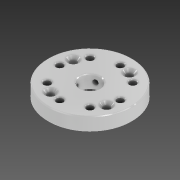
# Autodesk Inventor part: endeffector mount part
Saved by Autodesk Inventor 2020 (Build 240168000, 168)
## iProperties
Created: 2020-05-18
Part Number: endeffector mount part
Material: Generic
Document SubType Name: Modeling
Designer: stefa
Density: 1 g/cm^3
Appearance: Aluminum - Polished
Author: stefa
Autodesk Inventor part; units mm, degrees
ref_plane "YZ Plane" through (0, 0, 0) normal (1, 0, 0) x (0, 1, 0)
ref_plane "XZ Plane" through (0, 0, 0) normal (0, 1, 0) x (-1, 0, 0)
sketch "Sketch1" plane through (0, 0, 0) normal (0, 1, 0) x (-1, 0, 0)
  circle A0 centre (0, 0) radius 6
  circle A1 centre (0, 0) radius 25
  circle A2 centre (0, -18) radius 2
  circle A3 centre (12.7279, -12.7279) radius 2
  circle A4 centre (18, 0) radius 2
  circle A5 centre (12.7279, 12.7279) radius 2
  circle A6 centre (0, 18) radius 2
  circle A7 centre (-12.7279, 12.7279) radius 2
  circle A8 centre (-18, 0) radius 2
  circle A9 centre (-12.7279, -12.7279) radius 2
  circle A10 centre (16.682, -6.761) radius 2
  circle A11 centre (6.761, 16.682) radius 2
  circle A12 centre (-16.682, 6.761) radius 2
  circle A13 centre (-6.761, -16.682) radius 2
  dimension "d0" = 50
  dimension "d1" = 12
  dimension "d4" = 4
  dimension "d5" = 18
  dimension "d8" = 360
  dimension "d18" = 4
  dimension "d21" = 13.7766
  dimension "d22" = 6.8883
  dimension "d23" = 18
  dimension "d26" = 360
  constraints: 14 centre point, 2 coincident, 1 vertical alignment, 26 other
  measures "d0" diameter of A1
  measures "d1" diameter of A0
  measures "d4" diameter of A2
  measures "d5" distance of A2.centre point (0, 0)
  measures "d18" diameter of A10
  measures "d21" distance of A3.centre A4.centre
  measures "d22" distance of A10.centre A4.centre
  measures "d23" distance of A10.centre point (0, 0)
extrude "Extrusion1" add sketch "Sketch1" along normal blind 8
ref_plane "Work Plane2" through (0, 0, 0) normal (0.3826834, 0, 0.9238795) x (0, 1, 0)
sketch "Sketch2" plane through (0, 0, 0) normal (0.3826834, 0, 0.9238795) x (0, 1, 0)
  circle A0 centre (4, 0) radius 1.5
  line L0 (8, -25) -> (8, 25) projected
  line L1 (0, -25) -> (0, 25) projected
  point P0 (0, 0)
  dimension "d11" = 3
  dimension "d12" = 8
  dimension "d13" = 4
  constraints: 1 centre point
  measures "d11" diameter of A0
  measures "d12" distance between parallel lines of L0 L1
  measures "d13" distance from line of A0.centre L0
extrude "Extrusion2" cut sketch "Sketch2" against normal up to surface round surface about axis through (0, 0, 0) along (0, 1, 0) radius 25 far side no
thread "Thread1" size "M3x0.5" class "6H" standard "ANSI Metric M Profile" full length
chamfer "Chamfer1" distance 1.5 angle 45 4 edges at (18.682, 8, 6.761) (-4.761, 8, 16.682) (-14.682, 8, -6.761) (8.761, 8, -16.682)
thread "Thread2" size "M4x0.7" class "6H" standard "ANSI Metric M Profile" full length
thread "Thread3" size "M4x0.7" class "6H" standard "ANSI Metric M Profile" full length
thread "Thread4" size "M4x0.7" class "6H" standard "ANSI Metric M Profile" full length
thread "Thread5" size "M4x0.7" class "6H" standard "ANSI Metric M Profile" full length
thread "Thread6" size "M4x0.7" class "6H" standard "ANSI Metric M Profile" full length
thread "Thread7" size "M4x0.7" class "6H" standard "ANSI Metric M Profile" full length
thread "Thread8" size "M4x0.7" class "6H" standard "ANSI Metric M Profile" full length
thread "Thread9" size "M4x0.7" class "6H" standard "ANSI Metric M Profile" full length
chamfer "Chamfer2" distance 0.5 angle 45 25 edges at (25, 8, 0) (6, 8, 0) (25, 0, 0) (6, 0, 0) (14.7279, 8, -12.7279) (20, 8, 0) (14.7279, 8, 12.7279) (2, 8, 18) (-10.7279, 8, 12.7279) (-16, 8, 0) (-10.7279, 8, -12.7279) (2, 8, -18) (-10.0215, 2.5836, -22.9035) (2, 0, -18) (8.761, 0, -16.682) (14.7279, 0, -12.7279) (20, 0, 0) (18.682, 0, 6.761) (14.7279, 0, 12.7279) (2, 0, 18) (-4.761, 0, 16.682) (-10.7279, 0, 12.7279) (-16, 0, 0) (-14.682, 0, -6.761) (-10.7279, 0, -12.7279)
pattern_circular "Circular Pattern1" count 2 over 90 about axis through (0, -10, 0) along (0, 1, 0) of "Extrusion2"
equation "\"d22\" = 0.5 * d21"
equation "\"d13\" = 0.5 * d12"
body "Solid1"
